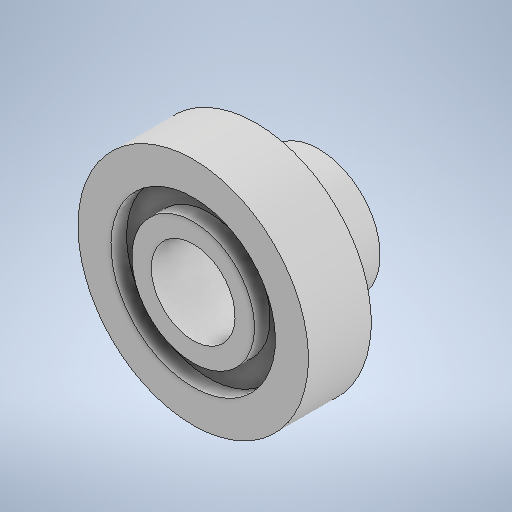
# Autodesk Inventor part: engrenage_simplifie_nouveau
Saved by Autodesk Inventor 2025.2 (Build 292293000, 293)
## iProperties
Created: 2025-05-05
Part Number: engrenage_simplifie_nouveau
Material: Générique
Document SubType Name: Modeling
Designer: enezl
Density: 1 g/cm^3
Appearance: Par défaut
Author: enezl
Autodesk Inventor part; units mm, degrees
ref_plane "YZ Plane" through (0, 0, 0) normal (1, 0, 0) x (0, 1, 0)
ref_plane "XZ Plane" through (0, 0, 0) normal (0, 1, 0) x (-1, 0, 0)
ref_plane "XY Plane" through (0, 0, 0) normal (0, 0, 1) x (1, 0, 0)
sketch "Esquisse1" plane through (0, 0, 0) normal (1, 0, 0) x (0, 1, 0)
  line L0 (0, 21.0755) -> (0, -24.2543)
  line L1 (7.85, -1.5) -> (7.85, 0)
  line L2 (7.85, 0) -> (11, 0)
  line L3 (11, 0) -> (11, -6)
  line L4 (11, -6) -> (7.85, -6)
  line L5 (7.85, -6) -> (7.85, -4.5)
  line L6 (7.85, -4.5) -> (5.85, -4.5)
  line L7 (5.85, -4.5) -> (5.85, -12)
  line L8 (5.85, -12) -> (4, -12)
  line L9 (7.85, -1.5) -> (5.85, -1.5)
  line L10 (5.85, -1.5) -> (5.85, 0)
  line L11 (5.85, 0) -> (4, 0)
  line L12 (4, 0) -> (4, -12)
  line L13 (6.85, -1.5) -> (6.85, -4.5) construction
  line L14 (6.85, -3) -> (11, -3) construction
  point P0 (0, 0)
  point P1 (7.85, -5.25)
  dimension "d0" = 11.7
  dimension "d1" = 8
  dimension "d2" = 12
  dimension "d3" = 6
  dimension "d4" = 22
  dimension "d5" = 2
  dimension "d6" = 3
  constraints: 30 end point, 8 perpendicular, 5 midpoint, 3 point on line, 2 collinear, 2 horizontal, 2 vertical
  measures "d0" diameter of L7 L0
  measures "d1" diameter of L12 L0
  measures "d2" distance of L11.end L8.end
  measures "d3" distance between parallel lines of L4 L11
  measures "d4" diameter of L3 L0
  measures "d5" distance from line of L7 point (7.85, -5.25)
  measures "d6" distance of L13.start L13.end
revolve "Révolution1" add sketch "Esquisse1" angle 360 about axis through (0, 0, 21.0755) along (0, 0, -1)
